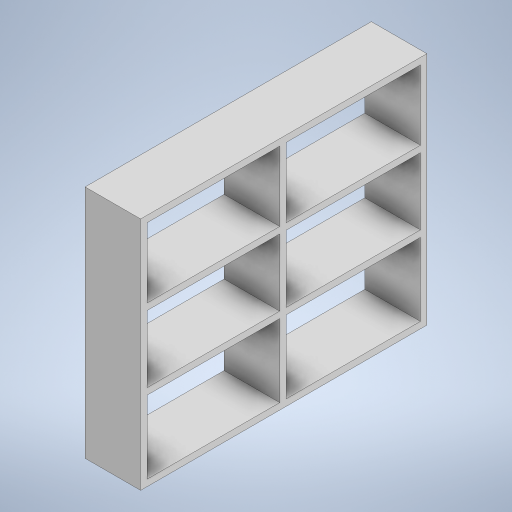
# Autodesk Inventor part: Estante
Saved by Autodesk Inventor 2023 (Build 270158000, 158)
## iProperties
Created: 2023-05-26
Part Number: Estante
Material: Genérico
Document SubType Name: Modeling
Designer: Valentina Cruz DP
Density: 1 g/cm^3
Appearance: Valor por defecto
Author: Valentina Cruz DP
Autodesk Inventor part; units mm, degrees
ref_plane "YZ Plane" through (0, 0, 0) normal (1, 0, 0) x (0, 1, 0)
ref_plane "XZ Plane" through (0, 0, 0) normal (0, 1, 0) x (-1, 0, 0)
ref_plane "XY Plane" through (0, 0, 0) normal (0, 0, 1) x (1, 0, 0)
sketch "Boceto1" plane through (0, 0, 0) normal (1, 0, 0) x (0, 1, 0)
  line L0 (0, 0) -> (436, 0)
  line L1 (436, 0) -> (436, -531)
  line L2 (436, -531) -> (0, -531)
  line L3 (0, -531) -> (0, 0)
  line L4 (0, -531) -> (12, -531)
  line L5 (12, -531) -> (12, 0)
  line L6 (12, 0) -> (0, 0)
  line L7 (0, 0) -> (0, -531)
  line L8 (436, -531) -> (424, -531)
  line L9 (424, -531) -> (424, -513.995)
  line L10 (436, -513.995) -> (436, -531)
  line L11 (436, 0) -> (424, 0)
  line L12 (424, 0) -> (424, -531)
  line L13 (424, -531) -> (436, -531)
  line L14 (436, -531) -> (436, 0)
  line L15 (0, 0) -> (436, 0)
  line L16 (436, 0) -> (436, -12)
  line L17 (436, -12) -> (0, -12)
  line L18 (0, -12) -> (0, 0)
  line L19 (0, -531) -> (436, -531)
  line L20 (436, -531) -> (436, -519)
  line L21 (436, -519) -> (0, -519)
  line L22 (0, -519) -> (0, -531)
  line L23 (12, -519) -> (147, -519)
  line L24 (147, -519) -> (147, -270)
  line L25 (147, -270) -> (12, -270)
  line L26 (12, -270) -> (12, -519)
  line L27 (12, -270) -> (424, -270)
  line L28 (424, -270) -> (424, -258)
  line L29 (424, -258) -> (12, -258)
  line L30 (12, -258) -> (12, -270)
  line L31 (147, -519) -> (159, -519)
  line L32 (159, -519) -> (159, -12)
  line L33 (159, -12) -> (147, -12)
  line L34 (147, -12) -> (147, -519)
  line L35 (159, -519) -> (283, -519)
  line L36 (283, -519) -> (283, -270)
  line L37 (283, -270) -> (159, -270)
  line L38 (159, -270) -> (159, -519)
  line L39 (283, -519) -> (295, -519)
  line L40 (295, -519) -> (295, -270)
  line L41 (295, -270) -> (283, -270)
  line L42 (283, -270) -> (283, -519)
  line L43 (295, -258) -> (295, -12)
  line L44 (283, -12) -> (283, -258)
  point P0 (424, -12)
  point P1 (159, -258)
  point P2 (159, -270)
  point P3 (12, -12)
  point P4 (147, -258)
  point P5 (424, -519)
  point P6 (424, -519)
  dimension "d0" = 436
  dimension "d1" = 531
  dimension "d2" = 12
  dimension "d3" = 12
  dimension "d4" = 12
  dimension "d5" = 12
  dimension "d6" = 12
  dimension "d7" = 135
  dimension "d8" = 249
  dimension "d9" = 12
  dimension "d10" = 12
  dimension "d11" = 124
  dimension "d12" = 12
  constraints: 90 end point, 21 parallel, 13 perpendicular, 13 point on line, 11 horizontal
  measures "d0" distance of L1.end L2.end
  measures "d1" distance of L0.end L1.end
  measures "d2" distance of L6.end L5.end
  measures "d3" distance of L9.end L10.start
  measures "d4" distance of L13.end L8.end
  measures "d5" distance of L15.end L16.end
  measures "d6" distance of L20.end L19.end
  measures "d7" distance of L25.end L24.end
  measures "d8" distance of L24.end L23.end
  measures "d9" distance of L28.end L27.end
  measures "d10" distance of L33.end L32.end
  measures "d11" distance of L37.end L36.end
  measures "d12" distance of L41.end L40.end
extrude "Extrusión2" add sketch "Boceto1" against normal blind 103 contours L0 L5 L17 L3 | L0 L12 L17 L5 | L17 L5 L21 L3 | L0 L1 L17 L12 | L21 L5 L2 L3 | L17 L1 L21 L9 L12 | L29 L34 L25 L5 | L17 L32 L29 L34 | L21 L9 L2 L5 | L12 L27 L32 L29 | L43 L29 L44 L17 | L29 L32 L27 L34 | L24 L27 L32 L21 | L9 L21 L1 L2 | L40 L21 L36 L27
